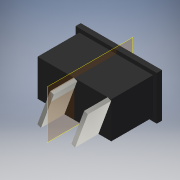
# Autodesk Inventor part: Switch
Saved by Autodesk Inventor 2018 (Build 220112000, 112)
## iProperties
Created: 2018-05-25
Part Number: Switch
Material: Generic
Document SubType Name: Modeling
Designer: Jasper
Density: 1 g/cm^3
Appearance: Default
Author: Jasper
Autodesk Inventor part; units mm, degrees
ref_plane "YZ Plane" through (0, 0, 0) normal (1, 0, 0) x (0, 1, 0)
ref_plane "XZ Plane" through (0, 0, 0) normal (0, 1, 0) x (-1, 0, 0)
ref_plane "XY Plane" through (0, 0, 0) normal (0, 0, 1) x (1, 0, 0)
sketch "Sketch1" plane through (0, 0, 0) normal (0, 1, 0) x (-1, 0, 0)
  line L0 (-14.3, 7.05) -> (14.3, 7.05)
  line L1 (14.3, 7.05) -> (14.3, -7.05)
  line L2 (14.3, -7.05) -> (-14.3, -7.05)
  line L3 (-14.3, -7.05) -> (-14.3, 7.05)
  line L4 (-14.3, 7.05) -> (14.3, -7.05) construction
  line L5 (14.3, 7.05) -> (-14.3, -7.05) construction
  point P0 (0, 0)
  dimension "d0" = 28.6
  dimension "d1" = 14.1
  constraints: 12 end point, 2 midpoint, 2 parallel, 1 horizontal, 1 perpendicular
  measures "d0" distance of L0.start L0.end
  measures "d1" distance of L0.end L1.end
extrude "Extrusion1" add sketch "Sketch1" along normal blind 16.2
sketch "Sketch2" plane through (0, 0, 0) normal (0, -1, 0) x (1, 0, 0)
  line L0 (9.3547, -7.05) -> (14.3, 6.537)
  line L1 (14.3, 6.537) -> (12.8905, 7.05)
  line L2 (12.8905, 7.05) -> (7.9452, -6.537)
  line L3 (7.9452, -6.537) -> (9.3547, -7.05)
  line L4 (9.3547, -7.05) -> (12.8905, 7.05) construction
  line L5 (14.3, 6.537) -> (7.9452, -6.537) construction
  line L6 (-14.3, -7.05) -> (-14.3, 7.05) construction
  line L7 (-14.3, 0) -> (14.3, 0) construction
  line L8 (14.3, 7.05) -> (14.3, -7.05) construction
  line L9 (14.3, 7.05) -> (-14.3, 7.05) construction
  line L10 (-14.3, -7.05) -> (14.3, -7.05) construction
  line L11 (14.3, -7.05) -> (14.3, 7.05) construction
  line L12 (-5.2548, -6.537) -> (-0.3095, 7.05)
  line L13 (-0.3095, 7.05) -> (1.1, 6.537)
  line L14 (1.1, 6.537) -> (-3.8453, -7.05)
  line L15 (-3.8453, -7.05) -> (-5.2548, -6.537)
  line L16 (-5.2548, -6.537) -> (1.1, 6.537) construction
  line L17 (-0.3095, 7.05) -> (-3.8453, -7.05) construction
  point P0 (0, 0)
  point P1 (11.1226, 0)
  point P2 (-2.0774, 0)
  dimension "d5" = 1.5
  dimension "d6" = 70
  dimension "d7" = 1.5
  dimension "d8" = 13.2
  constraints: 26 end point, 6 midpoint, 5 parallel, 5 point on line, 2 perpendicular
  measures "d5" distance between parallel lines of L0 L2
  measures "d6" angle of L7 L0
  measures "d7" distance between parallel lines of L14 L12
  measures "d8" distance of point (11.123, 0) point (-2.077, 0)
extrude "Extrusion2" add sketch "Sketch2" along normal blind 9.1 separate body
sketch "Sketch3" plane through (0, 16.2, 0) normal (0, 1, 0) x (1, 0, 0)
  line L0 (-15.75, -8.5) -> (15.75, -8.5)
  line L1 (15.75, -8.5) -> (15.75, 8.5)
  line L2 (15.75, 8.5) -> (-15.75, 8.5)
  line L3 (-15.75, 8.5) -> (-15.75, -8.5)
  line L4 (-15.75, -8.5) -> (15.75, 8.5) construction
  line L5 (15.75, -8.5) -> (-15.75, 8.5) construction
  point P0 (0, 0)
  dimension "d11" = 17
  dimension "d12" = 31.5
  constraints: 12 end point, 2 midpoint, 2 parallel, 1 horizontal, 1 perpendicular
  measures "d11" distance of L2.end L0.start
  measures "d12" distance of L1.end L2.end
extrude "Extrusion3" add sketch "Sketch3" along normal blind 2 bodies 1
sketch "Sketch4" plane through (0, 18.2, 0) normal (0, 1, 0) x (1, 0, 0)
  line L0 (12.75, -5.5) -> (-12.75, -5.5)
  line L1 (-12.75, -5.5) -> (-12.75, 5.5)
  line L2 (-12.75, 5.5) -> (12.75, 5.5)
  line L3 (12.75, 5.5) -> (12.75, -5.5)
  line L4 (12.75, -5.5) -> (-12.75, 5.5) construction
  line L5 (-12.75, -5.5) -> (12.75, 5.5) construction
  line L6 (-15.75, 8.5) -> (-15.75, -8.5) projected
  line L7 (-15.75, -8.5) -> (15.75, -8.5) projected
  point P0 (0, 0)
  dimension "d15" = 3
  dimension "d16" = 3
  constraints: 12 end point, 2 midpoint, 2 parallel, 1 horizontal, 1 perpendicular
  measures "d15" distance between parallel lines of L1 L6
  measures "d16" distance between parallel lines of L7 L0
extrude "Extrusion4" add sketch "Sketch4" along normal blind 2 bodies 1
sketch "Sketch5" plane through (0, 20.2, 0) normal (0, 1, 0) x (1, 0, 0)
  line L0 (-12.75, 5.5) -> (-12.75, -5.5) construction
  line L1 (-12.75, 0) -> (0, 0) construction
  line L2 (0, 0) -> (12.75, 0) construction
  line L3 (12.75, 5.5) -> (12.75, -5.5) construction
  circle A0 centre (-6.375, 0) radius 3
  circle A1 centre (-6.375, 0) radius 4
  line L4 (9.875, -0.5) -> (2.875, -0.5)
  line L5 (2.875, -0.5) -> (2.875, 0.5)
  line L6 (2.875, 0.5) -> (9.875, 0.5)
  line L7 (9.875, 0.5) -> (9.875, -0.5)
  line L8 (9.875, -0.5) -> (2.875, 0.5) construction
  line L9 (2.875, -0.5) -> (9.875, 0.5) construction
  point P0 (6.375, 0)
  dimension "d19" = 1
  dimension "d20" = 6
  dimension "d21" = 1
  dimension "d22" = 7
  constraints: 16 end point, 6 midpoint, 2 centre point, 2 horizontal, 2 parallel, 1 coincident, 1 perpendicular
  measures "d19" radial gap between concentric circles of A1 A0
  measures "d20" diameter of A0
  measures "d21" distance of L4.end L5.end
  measures "d22" distance of L5.end L6.end
extrude "Extrusion5" add sketch "Sketch5" along normal blind 1 separate body
ref_plane "Work Plane1" through (0, 0, 7.05) normal (1, 0, 0) x (0, 0, -1)
body "Solid1"
body "Solid2"
body "Solid3"
